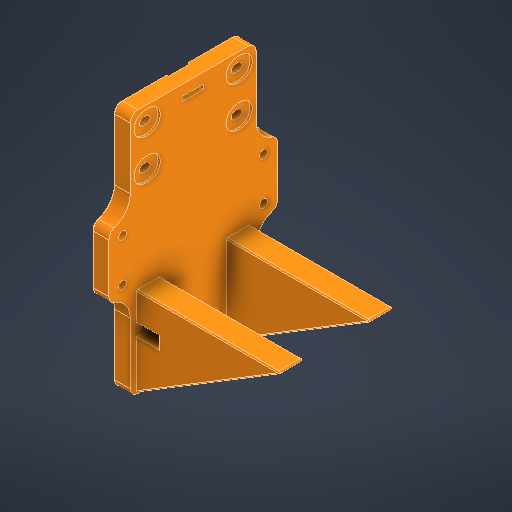
# Autodesk Inventor part: Soporte del primer segmento
Saved by Autodesk Inventor 2026 (Build 300175050, 175E)
## iProperties
Created: 2025-07-21
Part Number: Soporte del primer segmento
Material: Plastico PETG
Document SubType Name: Modeling
Designer: bello
Density: 1.27 g/cm^3
Appearance: Naranja
Author: bello
Autodesk Inventor part; units mm, degrees
ref_plane "YZ Plane" through (0, 0, 0) normal (1, 0, 0) x (0, 1, 0)
ref_plane "XZ Plane" through (0, 0, 0) normal (0, 1, 0) x (-1, 0, 0)
ref_plane "XY Plane" through (0, 0, 0) normal (0, 0, 1) x (1, 0, 0)
sketch "Boceto2" plane through (0, 0, 0) normal (1, 0, 0) x (0, 1, 0)
  line L0 (0, 0) -> (0, -36)
  arc A0 (-5, -41) -> (0, -36) centre (-5, -36) ccw
  line L1 (-5, -41) -> (-45, -41)
  arc A1 (-64.1, -55) -> (-59.1011, -51.5036) centre (-63.8713, -50.0052) ccw
  arc A2 (-45, -41) -> (-59.1011, -51.5036) centre (-44.7905, -55.9985) ccw
  line L2 (-64.1, -55) -> (-80.1, -55)
  line L3 (-80.1, -55) -> (-80.1, 0)
  line L4 (-80.1, 0) -> (0, 0)
  line L5 (-80.1, 0) -> (-160.2, 0)
  line L6 (0, 0) -> (0, 36)
  arc A3 (0, 36) -> (-5, 41) centre (-5, 36) ccw
  line L7 (-5, 41) -> (-45, 41)
  arc A4 (-59.1011, 51.5036) -> (-64.1, 55) centre (-63.8713, 50.0052) ccw
  arc A5 (-59.1011, 51.5036) -> (-45, 41) centre (-44.7905, 55.9985) ccw
  line L8 (-64.1, 55) -> (-80.1, 55)
  line L9 (-80.1, 55) -> (-80.1, 0)
  line L10 (-160.2, 0) -> (-160.2, -36)
  arc A6 (-160.2, -36) -> (-155.2, -41) centre (-155.2, -36) ccw
  line L11 (-155.2, -41) -> (-115.2, -41)
  arc A7 (-101.0989, -51.5036) -> (-96.1, -55) centre (-96.3287, -50.0052) ccw
  arc A8 (-101.0989, -51.5036) -> (-115.2, -41) centre (-115.4095, -55.9985) ccw
  line L12 (-96.1, -55) -> (-80.1, -55)
  arc A9 (-155.2, 41) -> (-160.2, 36) centre (-155.2, 36) ccw
  line L13 (-155.2, 41) -> (-115.2, 41)
  arc A10 (-96.1, 55) -> (-101.0989, 51.5036) centre (-96.3287, 50.0052) ccw
  arc A11 (-115.2, 41) -> (-101.0989, 51.5036) centre (-115.4095, 55.9985) ccw
  line L14 (-96.1, 55) -> (-80.1, 55)
  line L15 (-160.2, 0) -> (-160.2, 36)
  dimension "d0" = 36
  dimension "d5" = 5
  dimension "d22" = 40
  dimension "d26" = 5
  dimension "d27" = 15
  dimension "d99" = 16
  constraints: 32 end point, 26 symmetric about line, 24 point on circle, 12 centre point, 3 horizontal, 2 vertical, 1 perpendicular, 1 tangent, 10 other
  measures "d0" distance of L0.start L0.end
  measures "d5" radius of A0
  measures "d22" distance of L1.start L1.end
  measures "d26" radius of A1
  measures "d27" radius of A2
  measures "d99" distance of L2.start L2.end
extrude "Extrusión1" add sketch "Boceto2" along normal blind 11
sketch "Boceto3" plane through (0, 0, 0) normal (-1, 0, 0) x (0, 0, 1)
  line L0 (-41, -45) -> (-41, -5) projected
  line L1 (-7, -10) -> (7, -10)
  line L2 (7, -10) -> (7, -7)
  line L3 (7, -7) -> (-7, -7)
  line L4 (-7, -7) -> (-7, -10)
  line L5 (-7, -150.2) -> (7, -150.2)
  line L6 (7, -150.2) -> (7, -153.2)
  line L7 (7, -153.2) -> (-7, -153.2)
  line L8 (-7, -153.2) -> (-7, -150.2)
  line L9 (-36, 0) -> (36, 0) projected
  line L10 (36, -160.2) -> (-36, -160.2) projected
  line L11 (-41, -155.2) -> (-41, -115.2) projected
  point P0 (0, 0)
  dimension "d31" = 14
  dimension "d32" = 3
  dimension "d101" = 7
  dimension "d102" = 34
  dimension "d103" = 7
  dimension "d104" = 34
  dimension "d105" = 14
  dimension "d106" = 3
  constraints: 16 end point, 3 perpendicular, 2 parallel, 1 horizontal
  measures "d31" distance of L1.start L1.end
  measures "d32" distance of L1.end L2.end
  measures "d101" distance between parallel lines of L3 L9
  measures "d102" distance between parallel lines of L0 L4
  measures "d103" distance between parallel lines of L10 L7
  measures "d104" distance between parallel lines of L11 L8
  measures "d105" distance of L8.end L5.end
  measures "d106" distance of L5.end L7.start
extrude "Extrusión2" cut sketch "Boceto3" against normal blind 11
sketch "Boceto4" plane through (0, 0, 0) normal (-1, 0, 0) x (0, 0, 1)
  line L0 (-7, -7) -> (-7, -10) projected
  line L1 (-7, -7) -> (7, -7)
  line L2 (7, -7) -> (7, 0)
  line L3 (7, 0) -> (-7, 0)
  line L4 (-7, 0) -> (-7, -7)
  line L5 (-7, -153.2) -> (7, -153.2) projected
  line L6 (36, -160.2) -> (-36, -160.2) projected
  line L7 (-7, -153.2) -> (7, -153.2)
  line L8 (7, -153.2) -> (7, -160.2)
  line L9 (7, -160.2) -> (-7, -160.2)
  line L10 (-7, -160.2) -> (-7, -153.2)
  point P0 (0, 0)
  point P1 (7, -153.2)
  dimension "d35" = 14
  constraints: 16 end point, 4 parallel, 2 horizontal, 2 perpendicular, 1 point on line
  measures "d35" distance of L0.start L1.end
extrude "Extrusión3" cut sketch "Boceto4" against normal blind 2
sketch "Boceto5" plane through (0, 0, 0) normal (-1, 0, 0) x (0, 0, 1)
  line L0 (0, 0) -> (0, -155)
  line L1 (-31, -10) -> (-29, -10)
  line L2 (-31, -36.5) -> (-29, -36.5)
  arc A0 (-31, -7.5) -> (-31, -12.5) centre (-31, -10) ccw
  arc A1 (-31, -34) -> (-31, -39) centre (-31, -36.5) ccw
  arc A2 (-29, -12.5) -> (-29, -7.5) centre (-29, -10) ccw
  line L3 (-31, -7.5) -> (-29, -7.5)
  line L4 (-31, -12.5) -> (-29, -12.5)
  arc A3 (-29, -39) -> (-29, -34) centre (-29, -36.5) ccw
  line L5 (-31, -34) -> (-29, -34)
  line L6 (-31, -39) -> (-29, -39)
  line L7 (31, -10) -> (29, -10)
  line L8 (31, -36.5) -> (29, -36.5)
  arc A4 (31, -12.5) -> (31, -7.5) centre (31, -10) ccw
  arc A5 (31, -39) -> (31, -34) centre (31, -36.5) ccw
  arc A6 (29, -7.5) -> (29, -12.5) centre (29, -10) ccw
  line L9 (31, -7.5) -> (29, -7.5)
  line L10 (31, -12.5) -> (29, -12.5)
  arc A7 (29, -34) -> (29, -39) centre (29, -36.5) ccw
  line L11 (31, -34) -> (29, -34)
  line L12 (31, -39) -> (29, -39)
  circle A8 centre (-46, -66.1) radius 2.6
  line L13 (-55, -64.1) -> (-47.6613, -64.1)
  circle A9 centre (46, -66.1) radius 2.6
  line L14 (-41, -45) -> (-41, -5) projected
  line L15 (-81.3279, -80.1) -> (88.948, -80.1)
  line L16 (-31, -150.2) -> (-29, -150.2)
  line L17 (-31, -123.7) -> (-29, -123.7)
  arc A10 (-31, -147.7) -> (-31, -152.7) centre (-31, -150.2) ccw
  arc A11 (-31, -121.2) -> (-31, -126.2) centre (-31, -123.7) ccw
  arc A12 (-29, -152.7) -> (-29, -147.7) centre (-29, -150.2) ccw
  line L18 (-31, -152.7) -> (-29, -152.7)
  line L19 (-31, -147.7) -> (-29, -147.7)
  arc A13 (-29, -126.2) -> (-29, -121.2) centre (-29, -123.7) ccw
  line L20 (-31, -126.2) -> (-29, -126.2)
  line L21 (-31, -121.2) -> (-29, -121.2)
  line L22 (31, -121.2) -> (29, -121.2)
  arc A14 (29, -121.2) -> (29, -126.2) centre (29, -123.7) ccw
  line L23 (31, -126.2) -> (29, -126.2)
  arc A15 (31, -126.2) -> (31, -121.2) centre (31, -123.7) ccw
  line L24 (31, -147.7) -> (29, -147.7)
  line L25 (31, -150.2) -> (29, -150.2)
  arc A16 (29, -147.7) -> (29, -152.7) centre (29, -150.2) ccw
  line L26 (31, -152.7) -> (29, -152.7)
  arc A17 (31, -152.7) -> (31, -147.7) centre (31, -150.2) ccw
  line L27 (31, -123.7) -> (29, -123.7)
  circle A18 centre (-46, -94.1) radius 2.6
  line L28 (-55, -96.1) -> (-47.6613, -96.1)
  circle A19 centre (46, -94.1) radius 2.6
  dimension "d49" = 5.2
  dimension "d44" = 26.5
  dimension "d46" = 2.5
  dimension "d47" = 2.5
  dimension "d48" = 2
  dimension "d51" = 2
  dimension "d107" = 10
  constraints: 56 end point, 56 symmetric about line, 32 point on circle, 18 centre point, 16 coincident, 9 horizontal, 1 parallel, 1 tangent, 20 other
  measures "d44" distance of L1.start L2.start
  measures "d46" radius of A0
  measures "d47" radius of A1
  measures "d48" distance of L1.start L1.end
  measures "d51" distance from line of L13 point (-46, -66.1)
  measures "d107" distance from line of L14 L1.start
extrude "Extrusión4" cut sketch "Boceto5" against normal blind 11
sketch "Boceto6" plane through (0, 0, 0) normal (-1, 0, 0) x (0, 0, 1)
  arc A0 (-29, -12.5) -> (-29, -7.5) centre (-29, -10) ccw projected
  arc A1 (-29, -17.6) -> (-29, -2.4) centre (-29, -10) ccw
  arc A2 (-31, -7.5) -> (-31, -12.5) centre (-31, -10) ccw projected
  arc A3 (-31, -2.4) -> (-31, -17.6) centre (-31, -10) ccw
  line L0 (-31, -2.4) -> (-29, -2.4)
  line L1 (-29, -17.6) -> (-31, -17.6)
  arc A4 (-29, -39) -> (-29, -34) centre (-29, -36.5) ccw projected
  arc A5 (-29, -44.1) -> (-29, -28.9) centre (-29, -36.5) ccw
  arc A6 (-31, -34) -> (-31, -39) centre (-31, -36.5) ccw projected
  arc A7 (-31, -28.9) -> (-31, -44.1) centre (-31, -36.5) ccw
  line L2 (-31, -28.9) -> (-29, -28.9)
  line L3 (-29, -44.1) -> (-31, -44.1)
  arc A8 (29, -7.5) -> (29, -12.5) centre (29, -10) ccw
  arc A9 (29, -2.4) -> (29, -17.6) centre (29, -10) ccw
  arc A10 (31, -12.5) -> (31, -7.5) centre (31, -10) ccw
  arc A11 (31, -17.6) -> (31, -2.4) centre (31, -10) ccw
  line L4 (31, -2.4) -> (29, -2.4)
  line L5 (29, -17.6) -> (31, -17.6)
  arc A12 (29, -34) -> (29, -39) centre (29, -36.5) ccw
  arc A13 (29, -28.9) -> (29, -44.1) centre (29, -36.5) ccw
  arc A14 (31, -39) -> (31, -34) centre (31, -36.5) ccw
  arc A15 (31, -44.1) -> (31, -28.9) centre (31, -36.5) ccw
  line L6 (31, -28.9) -> (29, -28.9)
  line L7 (29, -44.1) -> (31, -44.1)
  line L8 (-77.9189, -80.1) -> (76.0726, -80.1)
  arc A16 (-29, -152.7) -> (-29, -147.7) centre (-29, -150.2) ccw
  arc A17 (-29, -157.8) -> (-29, -142.6) centre (-29, -150.2) ccw
  arc A18 (-31, -147.7) -> (-31, -152.7) centre (-31, -150.2) ccw
  arc A19 (-31, -142.6) -> (-31, -157.8) centre (-31, -150.2) ccw
  line L9 (-31, -157.8) -> (-29, -157.8)
  line L10 (-29, -142.6) -> (-31, -142.6)
  arc A20 (-29, -126.2) -> (-29, -121.2) centre (-29, -123.7) ccw
  arc A21 (-29, -131.3) -> (-29, -116.1) centre (-29, -123.7) ccw
  arc A22 (-31, -121.2) -> (-31, -126.2) centre (-31, -123.7) ccw
  arc A23 (-31, -116.1) -> (-31, -131.3) centre (-31, -123.7) ccw
  line L11 (-31, -131.3) -> (-29, -131.3)
  line L12 (-29, -116.1) -> (-31, -116.1)
  line L13 (31, -131.3) -> (29, -131.3)
  arc A24 (31, -126.2) -> (31, -121.2) centre (31, -123.7) ccw
  arc A25 (29, -121.2) -> (29, -126.2) centre (29, -123.7) ccw
  line L14 (29, -116.1) -> (31, -116.1)
  arc A26 (29, -116.1) -> (29, -131.3) centre (29, -123.7) ccw
  arc A27 (31, -131.3) -> (31, -116.1) centre (31, -123.7) ccw
  arc A28 (29, -142.6) -> (29, -157.8) centre (29, -150.2) ccw
  arc A29 (29, -147.7) -> (29, -152.7) centre (29, -150.2) ccw
  arc A30 (31, -152.7) -> (31, -147.7) centre (31, -150.2) ccw
  arc A31 (31, -157.8) -> (31, -142.6) centre (31, -150.2) ccw
  line L15 (29, -142.6) -> (31, -142.6)
  line L16 (31, -157.8) -> (29, -157.8)
  line L17 (0, 7.3278) -> (0, -171.4245)
  point P0 (0, 0)
  dimension "d54" = 7.6
  dimension "d55" = 7.6
  dimension "d56" = 7.6
  constraints: 60 point on circle, 50 symmetric about line, 36 end point, 28 centre point, 16 coincident, 3 horizontal, 2 parallel, 1 vertical, 16 other
  measures "d54" radius of A1
  measures "d55" radius of A5
  measures "d56" radius of A7
extrude "Extrusión5" cut sketch "Boceto6" against normal blind 1.5
sketch "Boceto7" plane through (11, 0, 0) normal (1, 0, 0) x (0, 0, -1)
  arc A0 (-29, -12.5) -> (-29, -7.5) centre (-29, -10) ccw
  arc A1 (-29, -17.6) -> (-29, -2.4) centre (-29, -10) ccw
  arc A2 (-31, -7.5) -> (-31, -12.5) centre (-31, -10) ccw
  arc A3 (-31, -2.4) -> (-31, -17.6) centre (-31, -10) ccw
  line L0 (-31, -2.4) -> (-29, -2.4)
  line L1 (-29, -17.6) -> (-31, -17.6)
  arc A4 (-29, -39) -> (-29, -34) centre (-29, -36.5) ccw
  arc A5 (-29, -44.1) -> (-29, -28.9) centre (-29, -36.5) ccw
  arc A6 (-31, -34) -> (-31, -39) centre (-31, -36.5) ccw
  arc A7 (-31, -28.9) -> (-31, -44.1) centre (-31, -36.5) ccw
  line L2 (-31, -28.9) -> (-29, -28.9)
  line L3 (-29, -44.1) -> (-31, -44.1)
  line L4 (0, 0) -> (0, -155)
  line L5 (31, -28.9) -> (29, -28.9)
  arc A8 (31, -39) -> (31, -34) centre (31, -36.5) ccw
  arc A9 (29, -34) -> (29, -39) centre (29, -36.5) ccw
  line L6 (29, -44.1) -> (31, -44.1)
  arc A10 (29, -28.9) -> (29, -44.1) centre (29, -36.5) ccw
  arc A11 (31, -44.1) -> (31, -28.9) centre (31, -36.5) ccw
  arc A12 (29, -2.4) -> (29, -17.6) centre (29, -10) ccw
  arc A13 (29, -7.5) -> (29, -12.5) centre (29, -10) ccw
  arc A14 (31, -12.5) -> (31, -7.5) centre (31, -10) ccw
  arc A15 (31, -17.6) -> (31, -2.4) centre (31, -10) ccw
  line L7 (29, -17.6) -> (31, -17.6)
  line L8 (31, -2.4) -> (29, -2.4)
  point P0 (0, 0)
  dimension "d59" = 7.6
  dimension "d60" = 7.6
  dimension "d61" = 7.6
  constraints: 34 point on circle, 25 symmetric about line, 18 end point, 16 centre point, 8 coincident, 2 horizontal, 2 parallel, 8 other
  measures "d59" radius of A1
  measures "d60" radius of A5
  measures "d61" radius of A7
extrude "Extrusión6" cut sketch "Boceto7" against normal blind 1.5
sketch "Boceto8" plane through (0, 0, 0) normal (-1, 0, 0) x (0, 0, 1)
  circle A0 centre (-13, -140.7) radius 2
  line L0 (-7, -160.2) -> (-36, -160.2) projected
  line L1 (-41, -155.2) -> (-41, -115.2) projected
  line L2 (0, 19.5154) -> (0, -187.5043)
  circle A1 centre (13, -140.7) radius 2
  point P0 (0, 0)
  dimension "d66" = 4
  dimension "d108" = 19.5
  dimension "d109" = 28
  constraints: 2 centre point, 2 end point, 1 symmetric about line, 1 vertical, 1 other
  measures "d66" diameter of A0
  measures "d108" distance from line of L0 A0.centre
  measures "d109" distance from line of L1 A0.centre
extrude "Extrusión7" cut sketch "Boceto8" against normal blind 11
sketch "Boceto9" plane through (11, 0, 0) normal (1, 0, 0) x (0, 0, -1)
  line L0 (-37, -101.2) -> (-21.5, -101.2)
  line L1 (-21.5, -101.2) -> (-21.5, -159.2)
  line L2 (-21.5, -159.2) -> (-37, -159.2)
  line L3 (-37, -159.2) -> (-37, -101.2)
  line L4 (0, -155) -> (0, 0)
  line L5 (37, -101.2) -> (21.5, -101.2)
  line L6 (21.5, -101.2) -> (21.5, -159.2)
  line L7 (21.5, -159.2) -> (37, -159.2)
  line L8 (37, -159.2) -> (37, -101.2)
  line L9 (-26.604, -146.05) -> (-24.208, -150.2)
  line L10 (-24.208, -150.2) -> (-26.604, -154.35)
  line L11 (-26.604, -154.35) -> (-31.396, -154.35)
  line L12 (-31.396, -146.05) -> (-26.604, -146.05)
  line L13 (-33.396, -146.05) -> (-28.604, -146.05)
  line L14 (-28.604, -154.35) -> (-33.396, -154.35)
  line L15 (-33.396, -154.35) -> (-35.792, -150.2)
  line L16 (-35.792, -150.2) -> (-33.396, -146.05)
  line L17 (26.604, -146.05) -> (24.208, -150.2)
  line L18 (24.208, -150.2) -> (26.604, -154.35)
  line L19 (26.604, -154.35) -> (31.396, -154.35)
  line L20 (31.396, -146.05) -> (26.604, -146.05)
  line L21 (33.396, -146.05) -> (28.604, -146.05)
  line L22 (28.604, -154.35) -> (33.396, -154.35)
  line L23 (33.396, -154.35) -> (35.792, -150.2)
  line L24 (35.792, -150.2) -> (33.396, -146.05)
  line L25 (-36, -160.2) -> (36, -160.2) projected
  arc A0 (-31, -147.7) -> (-31, -152.7) centre (-31, -150.2) ccw projected
  point P0 (-29, -150.2)
  point P1 (-29, -150.2)
  dimension "d71" = 58
  dimension "d72" = 15.5
  dimension "d85" = 8.3
  dimension "d110" = 1
  dimension "d111" = 0
  constraints: 50 end point, 14 symmetric about line, 4 equal length, 2 coincident, 1 collinear, 1 horizontal, 1 perpendicular, 1 vertical, 16 other
  measures "d71" distance of L0.end L1.end
  measures "d72" distance of L0.start L0.end
  measures "d85" distance between parallel lines of L11 L12
  measures "d110" distance between parallel lines of L25 L2
  measures "d111" distance of A0.centre point (-31, -150.2)
extrude "Extrusión8" add sketch "Boceto9" along normal blind 95
sketch "Boceto10" plane through (11, 0, 0) normal (1, 0, 0) x (0, 0, -1)
  line L0 (0, -155) -> (0, 0)
  line L1 (-24.208, -123.7) -> (-26.604, -127.85)
  line L2 (-26.604, -127.85) -> (-31.396, -127.85)
  line L3 (-31.396, -119.55) -> (-26.604, -119.55)
  line L4 (-26.604, -119.55) -> (-24.208, -123.7)
  line L5 (-31.396, -119.55) -> (-41, -119.55)
  line L6 (-31.396, -127.85) -> (-41, -127.85)
  line L7 (-41, -119.55) -> (-41, -127.85)
  line L8 (24.208, -123.7) -> (26.604, -127.85)
  line L9 (26.604, -127.85) -> (31.396, -127.85)
  line L10 (31.396, -119.55) -> (26.604, -119.55)
  line L11 (26.604, -119.55) -> (24.208, -123.7)
  line L12 (31.396, -119.55) -> (41, -119.55)
  line L13 (31.396, -127.85) -> (41, -127.85)
  line L14 (41, -119.55) -> (41, -127.85)
  point P0 (-36, -155)
  point P1 (-29, -123.7)
  point P2 (-29, -123.7)
  point P3 (29, -123.7)
  point P4 (29, -123.7)
  dimension "d115" = 8.3
  constraints: 30 end point, 9 symmetric about line, 1 horizontal, 1 parallel, 1 vertical, 8 other
  measures "d115" distance between parallel lines of L2 L3
extrude "Extrusión9" cut sketch "Boceto10" along normal blind 15
sketch "Boceto11" plane through (11, -159.2, 37) normal (0, 0, 1) x (1, 0, 0)
  line L0 (0, 58) -> (95, 58) projected
  line L1 (0, 0) -> (95, 0) projected
  line L2 (95, 58) -> (0, 0)
  line L3 (0, 0) -> (95, 0)
  line L4 (0, 9) -> (95, 9) projected
  line L5 (95, 0) -> (95, 58)
  point P0 (-11, 159.2)
  constraints: 6 end point, 1 parallel, 1 perpendicular
extrude "Extrusión10" cut sketch "Boceto11" against normal blind 95
sketch "Boceto12" plane through (11, 0, 0) normal (1, 0, 0) x (0, 0, -1)
  circle A0 centre (-13, -140.7) radius 2 projected
  line L0 (-10.8927, -137.05) -> (-8.7853, -140.7)
  line L1 (-8.7853, -140.7) -> (-10.8927, -144.35)
  line L2 (-10.8927, -144.35) -> (-15.1073, -144.35)
  line L3 (-15.1073, -144.35) -> (-17.2147, -140.7)
  line L4 (-17.2147, -140.7) -> (-15.1073, -137.05)
  line L5 (-15.1073, -137.05) -> (-10.8927, -137.05)
  circle A1 centre (13, -140.7) radius 2 projected
  line L6 (15.1073, -137.05) -> (17.2147, -140.7)
  line L7 (17.2147, -140.7) -> (15.1073, -144.35)
  line L8 (15.1073, -144.35) -> (10.8927, -144.35)
  line L9 (10.8927, -144.35) -> (8.7853, -140.7)
  line L10 (8.7853, -140.7) -> (10.8927, -137.05)
  line L11 (10.8927, -137.05) -> (15.1073, -137.05)
  line L12 (-7, -150.2) -> (7, -150.2) projected
  point P0 (0, 0)
  dimension "d88" = 7.3
  constraints: 24 end point, 2 coincident, 2 collinear, 1 parallel, 26 other
  measures "d88" distance between parallel lines of L2 L5
extrude "Extrusión11" cut sketch "Boceto12" against normal blind 3.2 contours L0 L1 L2 L3 L4 L5 | A1 | L6 L7 L8 L9 L10 L11
fillet "Empalme2" radius 0.8 10 edges at (58.5, -101.2, 37) (58.5, -101.2, 21.5) (106, -101.2, 29.25) (58.5, -130.2, 21.5) (58.5, -130.2, 37) (58.5, -101.2, -21.5) (58.5, -101.2, -37) (106, -101.2, -29.25) (58.5, -130.2, -21.5) (58.5, -130.2, -37)
chamfer "Chaflán3" distance 0.8 angle 45 26 edges at (0, 0, 21.5) (0, -1.4645, 39.5355) (0, -25, 41) (0, -53.7509, 43.969) (0, -61.0056, 54.1025) (0, -80.1, 55) (0, -106.4491, 43.969) (0, -99.1944, 54.1025) (0, -135.2, 41) (0, -158.7355, 39.5355) (0, -160.2, 21.5) (0, -155.2, 7) (0, -150.2, 0) (0, -155.2, -7) (0, -158.7355, -39.5355) (0, -135.2, -41) (0, -106.4491, -43.969) (0, -99.1944, -54.1025) (0, -80.1, -55) (0, -61.0056, -54.1025) (0, -53.7509, -43.969) (0, -25, -41) (0, -1.4645, -39.5355) (0, -5, -7) (0, -10, 0) (0, -5, 7)
